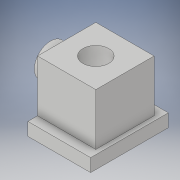
# Autodesk Inventor part: WackyPlug
Saved by Autodesk Inventor 2018.3 (Build 223284000, 284)
## iProperties
Created: 2020-01-21
Part Number: WackyPlug
Material: Generic
Document SubType Name: Modeling
Designer: 22perngrac
Density: 1 g/cm^3
Appearance: Default
Mass: 26.0699 g
Surface Area: 75.7385 cm^2
Volume: 26.0699 cm^3
Author: 22perngrac
Autodesk Inventor part; units mm, degrees
ref_plane "YZ Plane" through (0, 0, 0) normal (1, 0, 0) x (0, 1, 0)
ref_plane "XZ Plane" through (0, 0, 0) normal (0, 1, 0) x (-1, 0, 0)
ref_plane "XY Plane" through (0, 0, 0) normal (0, 0, 1) x (1, 0, 0)
sketch "Sketch1" plane through (0, 0, 0) normal (0, 1, 0) x (-1, 0, 0)
  line L0 (0, 0) -> (30.1625, 0)
  line L1 (30.1625, 0) -> (30.1625, -31.75)
  line L2 (30.1625, -31.75) -> (0, -31.75)
  line L3 (0, -31.75) -> (0, 0)
  dimension "d0" = 31.75
  dimension "d1" = 30.1625
  constraints: 8 end point, 2 parallel, 1 horizontal, 1 perpendicular
  measures "d0" distance of L0.end L1.end
  measures "d1" distance of L1.end L2.end
extrude "Extrusion1" add sketch "Sketch1" along normal blind 31.75
sketch "Sketch2" plane through (-30.1625, 0, 0) normal (0, 0, 1) x (1, 0, 0)
  line L0 (0, 0) -> (0, 31.75) projected
  line L1 (30.1625, 0) -> (30.1625, 31.75) projected
  line L2 (30.1625, 0) -> (0, 0) projected
  line L3 (0, 6.35) -> (30.1625, 6.35)
  line L4 (30.1625, 6.35) -> (30.1625, 31.75)
  line L5 (30.1625, 31.75) -> (0, 31.75)
  line L6 (0, 31.75) -> (0, 6.35)
  dimension "d5" = 6.35
  constraints: 8 end point, 2 parallel, 1 horizontal, 1 perpendicular, 1 point on line
  measures "d5" distance between parallel lines of L2 L3
extrude "Extrusion2" cut sketch "Sketch2" against normal blind 1.5875 contours L0 L5 L1 L3
sketch "Sketch3" plane through (0, 0, 0) normal (1, 0, 0) x (0, 0, -1)
  line L0 (1.5875, 31.75) -> (1.5875, 6.35) projected
  line L1 (31.75, 0) -> (31.75, 31.75) projected
  line L2 (1.5875, 6.35) -> (31.75, 6.35)
  line L3 (31.75, 6.35) -> (31.75, 31.75)
  line L4 (31.75, 31.75) -> (1.5875, 31.75)
  line L5 (1.5875, 31.75) -> (1.5875, 6.35)
  point P0 (0, 0)
  constraints: 8 end point, 2 parallel, 1 horizontal, 1 perpendicular
extrude "Extrusion3" cut sketch "Sketch3" against normal blind 1.5875
sketch "Sketch4" plane through (0, 0, -31.75) normal (0, 0, -1) x (-1, 0, 0)
  line L0 (0, 6.35) -> (30.1625, 6.35) projected
  line L1 (30.1625, 6.35) -> (30.1625, 31.75) projected
  line L2 (1.5875, 6.35) -> (30.1625, 6.35)
  line L3 (30.1625, 6.35) -> (30.1625, 31.75)
  line L4 (30.1625, 31.75) -> (1.5875, 31.75)
  line L5 (1.5875, 31.75) -> (1.5875, 6.35)
  line L6 (1.5875, 31.75) -> (1.5875, 6.35) projected
  point P0 (0, 0)
  dimension "d10" = 0
  constraints: 8 end point, 2 parallel, 1 horizontal, 1 perpendicular, 1 point on line
  measures "d10" distance between parallel lines of L6 L5
extrude "Extrusion4" cut sketch "Sketch4" against normal blind 1.5875
sketch "Sketch9" plane through (0, 31.75, 0) normal (0, 1, 0) x (1, 0, 0)
  line L0 (0, 31.75) -> (0, 0) projected
  line L1 (-30.1625, 31.75) -> (0, 31.75) projected
  point P0 (-15.875, 15.875)
  dimension "d23" = 15.875
  dimension "d24" = 15.875
  measures "d23" distance from line of L0 point (-15.875, 15.875)
  measures "d24" distance from line of L1 point (-15.875, 15.875)
hole "Hole1" at (-15.875, 31.75, -15.875) direction (0, -1, 0) diameter 12.7 end through all
sketch "Sketch10" plane through (-30.1625, 0, -31.75) normal (-1, 0, 0) x (0, 0, 1)
  circle A0 centre (15.875, 19.05) radius 7.9375
  line L0 (31.75, 0) -> (31.75, 6.35) projected
  line L1 (1.5875, 31.75) -> (30.1625, 31.75) projected
  line L2 (30.1625, 6.35) -> (30.1625, 31.75) projected
  dimension "d33" = 15.875
  dimension "d34" = 15.875
  constraints: 1 centre point
  measures "d33" diameter of A0
  measures "d34" distance from line of A0.centre L0
extrude "Extrusion6" add sketch "Sketch10" along normal blind 7.9375
sketch "Sketch12" plane through (0, 0, 0) normal (1, 0, 0) x (0, 0, -1)
  line L0 (31.75, 6.35) -> (0, 6.35) projected
  line L1 (0, 0) -> (0, 6.35) projected
  line L2 (31.75, 0) -> (0, 0) projected
  line L3 (31.75, 0) -> (31.75, 6.35) projected
extrude "Extrusion8" add sketch "Sketch12" along normal blind 0.635
sketch "Sketch13" plane through (-30.1625, 0, 0) normal (0, 0, 1) x (1, 0, 0)
  line L0 (0, 6.35) -> (30.7975, 6.35) projected
  line L1 (0, 0) -> (0, 6.35) projected
  line L2 (30.7975, 0) -> (0, 0) projected
  line L3 (30.7975, 6.35) -> (30.7975, 0) projected
  point P0 (30.1625, 0)
extrude "Extrusion9" add sketch "Sketch13" along normal blind 3.175
sketch "Sketch14" plane through (-30.1625, 0, -31.75) normal (0, 0, -1) x (-1, 0, 0)
  line L0 (0, 6.35) -> (-30.7975, 6.35) projected
  line L1 (-30.7975, 0) -> (-30.7975, 6.35) projected
  line L2 (0, 0) -> (-30.7975, 0) projected
  line L3 (0, 0) -> (0, 6.35) projected
  point P0 (-30.1625, 0)
extrude "Extrusion10" add sketch "Sketch14" along normal blind 3.175
equation "\"d24\" = d23"
body "Solid1"
